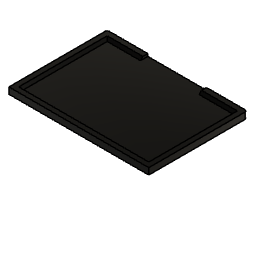
assembly_plate_hotel RevA (Autodesk Fusion 360 archive; units mm, degrees)
design "well_plate_tray"
Autodesk Fusion 360 part; units mm, degrees
sketch "Sketch1" plane through (0, 0, 0) normal (0, 0, 1) x (1, 0, 0)
  line L0 (71.5, -50.25) -> (-71.5, -50.25)
  line L1 (-71.5, -50.25) -> (-71.5, 50.25)
  line L2 (-71.5, 50.25) -> (71.5, 50.25)
  line L3 (71.5, 50.25) -> (71.5, -50.25)
  line L4 (71.5, -50.25) -> (-71.5, 50.25) construction
  line L5 (-71.5, -50.25) -> (71.5, 50.25) construction
  dimension "d4" = 143
  dimension "d5" = 100.5
  constraint horizontal L0
  constraint perpendicular L0 L1
  constraint parallel L0 L2
  constraint parallel L1 L3
  constraint coincident L4 origin
  constraint coincident L5 origin
  measures "d4" distance of L1.end L2.end
  measures "d5" distance of L0.end L1.end
extrude "Extrude1" add sketch "Sketch1" along normal blind 4
sketch "Sketch2" plane through (0, 0, 4) normal (0, 0, 1) x (-1, 0, 0)
  line L0 (-71.5, -50.25) -> (71.5, -50.25)
  line L1 (71.5, -50.25) -> (71.5, 50.25)
  line L2 (71.5, 50.25) -> (-71.5, 50.25)
  line L3 (-71.5, 50.25) -> (-71.5, -50.25)
  line L4 (-66.5, 45.25) -> (-66.5, -45.25)
  line L5 (-66.5, -45.25) -> (66.5, -45.25)
  line L6 (66.5, -45.25) -> (66.5, 45.25)
  line L7 (66.5, 45.25) -> (-66.5, 45.25)
extrude "Extrude2" add sketch "Sketch2" along normal blind 2.5
chamfer "Chamfer1" distance 2.5 angle 45 1 faces at (-22.1667, 15.0833, 4)
sketch "Sketch8" plane through (0, 0, 0) normal (0, 0, -1) x (1, 0, 0)
  line L0 (-71.5, -50.25) -> (71.5, -50.25)
  line L1 (71.5, -50.25) -> (71.5, 50.25)
  line L2 (71.5, 50.25) -> (-71.5, 50.25)
  line L3 (-71.5, 50.25) -> (-71.5, -50.25)
  line L4 (-15, -50.25) -> (15, -50.25)
  line L5 (15, -50.25) -> (15, -46.25)
  line L6 (15, -46.25) -> (-15, -46.25)
  line L7 (-15, -46.25) -> (-15, -50.25)
  line L8 (-15, -50.25) -> (15, -46.25) construction
  line L9 (15, -50.25) -> (-15, -46.25) construction
  line L10 (-15, -50.25) -> (-19, -50.25)
  line L11 (-19, -50.25) -> (-19, -15.25)
  line L12 (-19, -15.25) -> (-15, -15.25)
  line L13 (-15, -15.25) -> (-15, -50.25)
  line L14 (15, -50.25) -> (19, -50.25)
  line L15 (19, -50.25) -> (19, -15.25)
  line L16 (19, -15.25) -> (15, -15.25)
  line L17 (15, -15.25) -> (15, -50.25)
  point P0 (0, -48.25)
  dimension "d32" = 4
  dimension "d33" = 30
  dimension "d43" = 35
  dimension "d44" = 4
  constraint horizontal L4
  constraint perpendicular L4 L5
  constraint parallel L4 L6
  constraint parallel L5 L7
  constraint coincident L8 P0
  constraint coincident L9 P0
  constraint vertical origin P0
  constraint horizontal L10
  constraint vertical L11
  constraint horizontal L12
  constraint vertical L13
  constraint horizontal L14
  constraint vertical L15
  constraint horizontal L16
  constraint vertical L17
  constraint collinear L12 L16
  constraint equal L12 L16
  constraint collinear L0 L4
  measures "d32" distance of L4.end L5.end
  measures "d33" distance of L4.start L4.end
  measures "d43" distance of L10.end L11.end
  measures "d44" distance of L11.end L12.end
extrude "Extrude5" add sketch "Sketch8" along normal blind 45 contours L0 L7 L10 L11 L12 L13 | L0 L4 L5 L6 L7 L13 L17 | L0 L5 L14 L15 L16 L17
sketch "Sketch9" plane through (0, 46.25, 0) normal (0, -1, 0) x (1, 0, 0)
  line L0 (15, 0) -> (-15, 0)
  line L1 (-15, -45) -> (15, -45)
  line L2 (-71.5, 6.5) -> (71.5, 6.5)
  line L3 (0, 6.5) -> (0, -11)
  line L4 (0, -11) -> (0, -36)
  line L5 (-15, 0) -> (-15, -45)
  line L6 (15, -45) -> (15, 0)
  point P0 (0, -11)
  point P1 (0, -36)
  dimension "d36" = 25
  dimension "d37" = 17.5
  constraint midpoint L2 L3.start
  constraint perpendicular L0 L3
  constraint perpendicular L0 L4
  constraint coincident P0 L3.end
  constraint coincident P1 L4.end
  measures "d36" distance of P0 P1
  measures "d37" distance of L3.start P0
hole "Hole3" at (0, 46.25, -11) at (0, 46.25, -36) direction (0, 1, 0) diameter 6.6 depth 25 tip angle 118 countersink diameter 12.6 countersink angle 90
sketch "Sketch10" plane through (19, 0, 0) normal (1, 0, 0) x (0, 1, 0)
  line L0 (50.25, 0) -> (15.25, 0)
  line L1 (15.25, 0) -> (15.25, -45)
  line L2 (15.25, -45) -> (50.25, -45)
  line L3 (50.25, -45) -> (50.25, 0)
  ellipse E0 centre (15.25, -45) end of major axis (15.25, 0) minor radius 31
  line L4 (15.25, -90) -> (15.25, 0) construction
  line L5 (46.25, -45) -> (-15.75, -45) construction
  point P0 (46.25, -45)
  constraint coincident E0 L4.start
  constraint coincident E0 L0.end
  constraint coincident E0 P0
  constraint coincident E0 L5.end
  constraint coincident L1.end L2.start
  constraint perpendicular L2 L4
  constraint coincident P0 L5.start
  constraint coincident L0.end L1.start
extrude "Extrude6" cut sketch "Sketch10" against normal through all contours L1 L2 E0 | L1 L2 E0
sketch "Sketch11" plane through (0, 0, 6.5) normal (0, 0, 1) x (-1, 0, 0)
  line L0 (-66.5, 45.25) -> (66.5, 45.25)
  line L1 (66.5, 45.25) -> (66.5, -45.25)
  line L2 (66.5, -45.25) -> (-66.5, -45.25)
  line L3 (-66.5, -45.25) -> (-66.5, 45.25)
  line L4 (-71.5, 50.25) -> (-71.5, -50.25)
  line L5 (-71.5, -50.25) -> (71.5, -50.25)
  line L6 (71.5, -50.25) -> (71.5, 50.25)
  line L7 (71.5, 50.25) -> (-71.5, 50.25)
  line L8 (-30, -50.25) -> (30, -50.25)
  line L9 (30, -50.25) -> (30, -42.75)
  line L10 (30, -42.75) -> (-30, -42.75)
  line L11 (-30, -42.75) -> (-30, -50.25)
  line L12 (-30, -50.25) -> (30, -42.75) construction
  line L13 (30, -50.25) -> (-30, -42.75) construction
  line L14 (64, -42.75) -> (-64, -42.75)
  point P0 (0, -46.5)
  dimension "d47" = 60
  constraint horizontal L8
  constraint perpendicular L8 L9
  constraint parallel L8 L10
  constraint parallel L9 L11
  constraint coincident L12 P0
  constraint coincident L13 P0
  constraint coincident L5 L8.start
  constraint collinear L10 L14
  constraint vertical origin P0
  measures "d47" distance of L8.start L8.end
extrude "Extrude7" cut sketch "Sketch11" against normal up to surface (2.5 mm away) contours L2 L9 L10 L11 L14 | L2 L5 L8 L9 L11
fillet "Fillet1" radius 5 4 edges at (19, 32.75, 0) (15, 30.75, 0) (-15, 30.75, 0) (-19, 32.75, 0)
fillet "Fillet1" radius 2 2 edges at (71.5, 50.25, 3.25) (-71.5, 50.25, 3.25)
equation "well_plate_width = 85.5 mm"
equation "well_plate_length = 128 mm"
equation "well_plate_offset = 5 mm"
equation "d4 = well_plate_length + 3 * well_plate_offset"
equation "d5 = well_plate_width + 3 * well_plate_offset"
equation "d8 = -well_plate_offset"

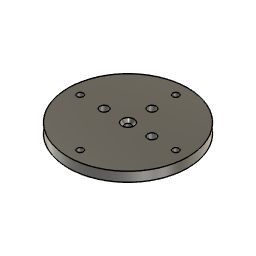
design "plate_hotel_base"
Autodesk Fusion 360 part; units mm, degrees
sketch "Sketch3" plane through (0, 0, 0) normal (0, 0, 1) x (1, 0, 0)
  circle A0 centre (0, 0) radius 62.5
  dimension "d12" = 125
  constraint coincident A0.centre origin
  measures "d12" diameter of A0
extrude "Extrude2" add sketch "Sketch3" along normal blind 10
sketch "Sketch4" plane through (0, 0, 10) normal (0, 0, 1) x (-1, 0, 0)
  circle A0 centre (0, 0) radius 62.5
  line L0 (0, 0) -> (0, -25)
  line L1 (0, -25) -> (0, -50)
  line L2 (0, 0) -> (25, 0)
  line L3 (25, 0) -> (50, 0)
  line L4 (0, 0) -> (-25, 0)
  line L5 (-25, 0) -> (-50, 0)
  line L6 (0, 0) -> (0, 25)
  line L7 (0, 25) -> (0, 50)
  point P0 (-25, 0)
  point P1 (25, 0)
  point P2 (0, -25)
  point P3 (0, -50)
  point P4 (-50, 0)
  point P5 (50, 0)
  point P6 (0, 50)
  point P7 (0, 25)
  dimension "d15" = 25
  constraint coincident A0.centre L0.start
  constraint collinear A0.centre P2 P6
  constraint collinear A0.centre P2 P3
  constraint coincident P2 L0.end
  constraint coincident P3 L1.end
  constraint parallel L0 L1
  constraint coincident P1 L2.end
  constraint horizontal L2
  constraint coincident P5 L3.end
  constraint parallel L2 L3
  constraint coincident P0 L4.end
  constraint parallel L2 L4
  constraint coincident P4 L5.end
  constraint parallel L2 L5
  constraint equal L0 L1
  constraint equal L4 L5
  constraint equal L2 L3
  constraint equal L2 L4
  constraint vertical L0
  constraint perpendicular L2 L6
  constraint coincident P6 L7.end
  constraint perpendicular L2 L7
  constraint coincident P7 L6.end
  constraint equal L0 L6
  constraint equal L6 L7
  constraint equal L0 L2
  measures "d15" distance of P1 P5
hole "Hole2" at (25, 0, 10) at (-25, 0, 10) at (0, 25, 10) direction (0, 0, -1) diameter 8.8646 end through all
hole "Hole3" at (0, 50, 10) at (50, 0, 10) at (0, -50, 10) at (-50, 0, 10) direction (0, 0, -1) diameter 6.4 end through all
hole "Hole4" at (0, 0, 10) direction (0, 0, -1) diameter 6.4 end through all countersink diameter 12.6 countersink angle 90
sketch "Sketch5" plane through (0, 0, 0) normal (0, 0, -1) x (1, 0, 0)
  circle A0 centre (0, 0) radius 3.2
  circle A1 centre (0, 50) radius 3.2
  circle A2 centre (0, -50) radius 3.2
  circle A3 centre (50, 0) radius 3.2
  circle A4 centre (-50, 0) radius 3.2
  circle A5 centre (25, 0) radius 4.4323
  circle A6 centre (-25, 0) radius 4.4323
  circle A7 centre (0, 0) radius 62.5
  line L0 (0, 0) -> (11.5, 0) construction
  line L1 (11.5, 0) -> (14.5, 0) construction
  line L2 (11.5, -3.125) -> (14.5, -3.125)
  line L3 (11.5, 3.125) -> (14.5, 3.125)
  line L4 (14.5, -3.125) -> (14.5, 3.125)
  line L5 (11.5, -3.125) -> (11.5, 3.125)
  circle A8 centre (0, -25) radius 4.4323
  line L6 (3.125, 11.5) -> (-3.125, 11.5)
  line L7 (3.125, 14.5) -> (-3.125, 14.5)
  line L8 (-3.125, 11.5) -> (-3.125, 14.5)
  line L9 (0, 11.5) -> (0, 14.5) construction
  line L10 (3.125, 11.5) -> (3.125, 14.5)
  line L11 (0, 0) -> (0, 11.5) construction
  line L12 (-11.5, 3.125) -> (-11.5, -3.125)
  line L13 (-14.5, 3.125) -> (-14.5, -3.125)
  line L14 (-11.5, -3.125) -> (-14.5, -3.125)
  line L15 (-11.5, 0) -> (-14.5, 0) construction
  line L16 (-11.5, 3.125) -> (-14.5, 3.125)
  line L17 (0, 0) -> (-11.5, 0) construction
  line L18 (-3.125, -11.5) -> (3.125, -11.5)
  line L19 (-3.125, -14.5) -> (3.125, -14.5)
  line L20 (3.125, -11.5) -> (3.125, -14.5)
  line L21 (0, -11.5) -> (0, -14.5) construction
  line L22 (-3.125, -11.5) -> (-3.125, -14.5)
  line L23 (0, 0) -> (0, -11.5) construction
  point P0 (0, 25)
  point P1 (-25, 0)
  point P2 (0, -25)
  dimension "d28" = 3
  dimension "d29" = 11.5
  dimension "d30" = 3.125
  dimension "d31" = -3.125
  dimension "d37" = 360
  constraint coincident A0.centre A7.centre
  constraint horizontal L0
  constraint parallel L0 L1
  constraint perpendicular L3 L4
  constraint perpendicular L3 L5
  constraint coincident L0.end L5
  constraint coincident L1.end L4
  measures "d28" distance of L0.end L1.end
  measures "d29" distance of A0.centre L0.end
extrude "Extrude3" cut sketch "Sketch5" against normal blind 3 contours L2 L3 L4 L5 | L12 L13 L14 L16 | L18 L19 L20 L22
equation "thickness = 15 mm"
equation "height = 60 mm"
equation "hole_hole_dist = 25 mm"
equation "d30 = ( 6.25 / 2 ) * 1 mm"
equation "d31 = -d30"
